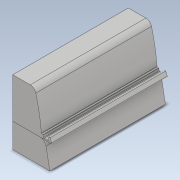
# Autodesk Inventor part: 0 零件
Saved by Autodesk Inventor 2022 (Build 260153000, 153)
## iProperties
Created: 2020-11-03
Part Number: 0 零件
Material: 一般
Document SubType Name: Modeling
Designer: p2013
Density: 1 g/cm^3
Appearance: 預設
Mass: 2999.3 g
Surface Area: 2074.78 cm^2
Volume: 2999.3 cm^3
Author: p2013
Autodesk Inventor part; units mm, degrees
ref_plane "YZ Plane" through (0, 0, 0) normal (1, 0, 0) x (0, 1, 0)
ref_plane "XZ Plane" through (0, 0, 0) normal (0, 1, 0) x (-1, 0, 0)
ref_plane "XY Plane" through (0, 0, 0) normal (0, 0, 1) x (1, 0, 0)
sketch "草圖1" plane through (0, 0, 0) normal (0, 0, 1) x (1, 0, 0)
  line L0 (0, 0) -> (-9.6483, 0) construction
  line L1 (0, 0) -> (0, 8.3837) construction
  line L2 (-7.5155, 4.4979) -> (-7.5, 11.3039)
  arc A0 (-4.2366, 11.9677) -> (-7.5, 11.3039) centre (-5.8, 11.3) ccw
  line L3 (-4.2366, 11.9677) -> (-0.1366, 2.3677)
  arc A1 (-3.1931, 0.8871) -> (-0.1366, 2.3677) centre (-1.7, 1.7) ccw
  line L4 (-3.1931, 0.8871) -> (-4.6931, 0.8871)
  line L5 (-4.6931, 0.8871) -> (-6.6931, 0)
  line L6 (-6.6931, 0) -> (-19.3096, 0)
  line L7 (-19.3096, 0) -> (-21.6815, 0.8871)
  line L8 (-21.6815, 0.8871) -> (-100.9388, 0.8871)
  line L9 (-21.0255, 4.4056) -> (-22.2246, 8.8809)
  line L10 (-22.8675, 9.5685) -> (-25.8843, 10.598)
  arc A2 (-22.2246, 8.8809) -> (-22.8675, 9.5685) centre (-23.1905, 8.6221) ccw
  line L11 (-13.2, 16.4786) -> (-10.2, 16.4786) construction
  line L12 (-10.2, 16.4786) -> (-10.2, 4.7787) construction
  line L13 (-10.2, 4.7787) -> (-13.2, 4.7787) construction
  line L14 (-13.2, 4.7787) -> (-13.2, 16.4786) construction
  arc A3 (-26.5573, 11.4548) -> (-44.0636, 105.2211) centre (-528.3565, -33.7147) ccw
  arc A4 (-26.5573, 11.4548) -> (-25.8843, 10.598) centre (-25.5613, 11.5444) ccw
  line L15 (-44.0636, 105.2211) -> (-100.9388, 105.2211)
  line L16 (-100.9388, 105.2211) -> (-100.9388, 0.8871)
  line L17 (-9.2215, 13) -> (-2.2458, 13) construction
  line L18 (-7.985, 4) -> (-19.485, 3.2966)
  arc A5 (-7.985, 4) -> (-7.5155, 4.4979) centre (-8.0155, 4.4991) ccw
  arc A6 (-21.0255, 4.4056) -> (-19.485, 3.2966) centre (-19.5766, 4.7938) ccw
  point P0 (-26.4995, 10.808)
  point P1 (-11.7, 4.7787)
  point P2 (-20.814, 3.6164)
  dimension "d0" = 13
  dimension "d4" = 1.7
  dimension "d5" = 1.7
  dimension "d9" = 1
  dimension "d13" = 3
  dimension "d14" = 10
  dimension "d25" = 1
  dimension "d28" = 2
  dimension "d29" = 1.5
  dimension "d31" = 7.5
  dimension "d35" = 23.257
  dimension "d37" = 3.5
  dimension "d38" = 0.5
  dimension "d39" = 11.5
  dimension "d40" = 9
  dimension "d41" = 1.5
  dimension "d53" = 503.8281
  dimension "d55" = 101.5
  dimension "d56" = 0.8871
  dimension "d57" = 12.6165
  dimension "d58" = 79.2574
  dimension "d59" = 20.507
  dimension "d60" = 104.3339
  dimension "d61" = 123.844
  dimension "d62" = 5.5417
  dimension "d63" = 8.6034
  dimension "d64" = 34.6018
  constraints: 39 end point, 15 point on circle, 14 tangent, 7 centre point, 5 horizontal, 5 point on line, 3 parallel, 2 perpendicular, 1 midpoint, 1 vertical
  measures "d4" radius of A0
  measures "d5" radius of A1
  measures "d9" radius of A2
  measures "d13" distance of L11.start L11.end
  measures "d14" horizontal distance of A1.centre point (-11.7, 4.779)
  measures "d25" radius of A4
  measures "d28" horizontal distance of L4.end L5.end
  measures "d29" distance of L4.start L4.end
  measures "d31" distance from line of L2.end L1
  measures "d35" angle of L3 L2
  measures "d37" angle of L6 L18
  measures "d38" radius of A5
  measures "d39" horizontal distance of L18.start L18.end
  measures "d40" distance from line of L17 L18.start
  measures "d41" radius of A6
  measures "d53" radius of A3
  measures "d55" angle of L18 L9
  measures "d56" distance between parallel lines of L8 L6
  measures "d57" distance of L5.end L6.end
  measures "d58" distance of L7.end L8.end
  measures "d59" angle of L8 L7
  measures "d60" distance of L15.end L8.end
  measures "d61" angle of L9 L10
  measures "d62" distance from line of L18 A2.centre
  measures "d63" distance from line of L18 A4.centre
  measures "d64" distance from line of L8 A3.centre
extrude "擠出1" add sketch "草圖1" along normal mid plane 300
fillet "圓角2" radius 3 3 edges at (-3.1931, 0.8871, 0) (-6.6931, 0, 0) (-4.6931, 0.8871, 0)
sketch "草圖4" plane through (0, 0, 0) normal (0, 0, 1) x (1, 0, 0)
  line L0 (-100.9388, 0.8871) -> (-29.2228, 0.8871)
  arc A0 (-14.4798, -11.3483) -> (-29.2228, 0.8871) centre (-29.2228, -14.1129) ccw
  line L1 (-14.4798, -11.3483) -> (-4.819, -62.867)
  line L2 (-100.9388, 0.8871) -> (-21.6815, 0.8871) projected
  line L3 (-4.819, -62.867) -> (-100.9388, -62.867)
  line L4 (-100.9388, -62.867) -> (-100.9388, 0.8871)
  point P0 (0, 0)
  dimension "d45" = 100.621
  dimension "d46" = 0
  dimension "d48" = 15
  dimension "d66" = 96.1198
  dimension "d67" = 63.7541
  constraints: 8 end point, 2 horizontal, 2 point on circle, 2 tangent, 1 centre point, 1 coincident, 1 perpendicular
  measures "d45" angle of L0 L1
  measures "d46" distance between parallel lines of L2 L0
  measures "d48" radius of A0
  measures "d66" distance of L1.end L3.end
  measures "d67" distance of L3.end L0.start
extrude "擠出2" add sketch "草圖4" along normal mid plane 300 separate body
fillet "圓角3" radius 15 1 edges at (-44.0636, 105.2211, 0)
